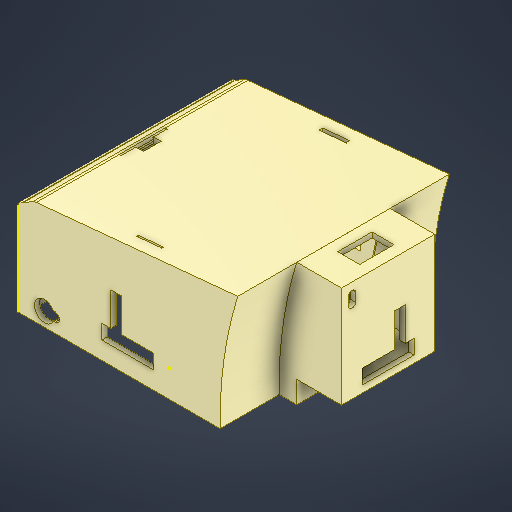
# Autodesk Inventor part: Tapa V.2
Saved by Autodesk Inventor 2026.2 (Build 302298010, 298A)
## iProperties
Created: 2026-05-06
Part Number: Tapa V.2
Material: Genérico
Document SubType Name: Modeling
Designer: migue
Density: 1 g/cm^3
Appearance: Nilón 6
Author: migue
Autodesk Inventor part; units mm, degrees
ref_plane "YZ Plane" through (0, 0, 0) normal (1, 0, 0) x (0, 1, 0)
ref_plane "XZ Plane" through (0, 0, 0) normal (0, 1, 0) x (-1, 0, 0)
sketch "Boceto1" plane through (0, 0, 0) normal (0, 1, 0) x (-1, 0, 0)
  line L0 (-38.316, 43.1554) -> (-63.666, 43.1554)
  line L1 (-63.666, 43.1554) -> (-63.666, -9.8446)
  line L2 (-63.666, -9.8446) -> (-38.316, -9.8446)
  line L3 (-72.7588, 16.6554) -> (45.2156, 16.6554) construction
  line L4 (-38.316, 76.6554) -> (86.334, 76.6554)
  line L5 (86.334, 76.6554) -> (86.334, -43.3446)
  line L6 (86.334, -43.3446) -> (-38.316, -43.3446)
  line L7 (-38.316, -43.3446) -> (-38.316, -9.8446)
  line L8 (-38.316, 43.1554) -> (-38.316, 76.6554)
  circle A0 centre (-42.216, 33.1554) radius 1.65
  circle A1 centre (-42.216, 0.1554) radius 1.65
  line L9 (83.334, 73.6554) -> (-35.316, 73.6554)
  line L10 (-35.316, -40.3446) -> (83.334, -40.3446)
  line L11 (83.334, -40.3446) -> (83.334, 73.6554)
  line L12 (-35.316, 73.6554) -> (-35.316, -40.3446)
  point P0 (-63.666, 16.6554)
  point P1 (-63.666, 16.6554)
  dimension "d5" = 53
  dimension "d6" = 120
  dimension "d7" = 124.65
  dimension "d8" = 25.35
  dimension "d9" = 33.5
  dimension "d10" = 3.3
  dimension "d11" = 16.5
  dimension "d12" = 3.9
  dimension "d13" = 3
  constraints: 26 end point, 6 parallel, 3 horizontal, 3 perpendicular, 2 centre point, 1 coincident, 1 midpoint, 1 symmetric about line, 1 vertical, 2 other
  measures "d5" distance of L2.start L0.end
  measures "d6" distance of L5.start L6.start
  measures "d7" distance of L6.start L7.start
  measures "d8" distance of L2.start L7.end
  measures "d9" distance between parallel lines of L0 L4
  measures "d10" diameter of A0
  measures "d11" distance from line of L3 A0.centre
  measures "d12" distance from line of A0.centre L8
  measures "d13" distance between parallel lines of L4 L9
extrude "Extrusión9" add sketch "Boceto1" against normal blind 3
sketch "Boceto4" plane through (0, 0, 0) normal (0, 1, 0) x (1, 0, 0)
  line L0 (-86.334, 43.3446) -> (38.316, 43.3446) projected
  line L1 (38.316, 43.3446) -> (-86.334, 43.3446)
  line L2 (-86.334, 43.3446) -> (-86.334, -76.6554)
  line L3 (-86.334, -76.6554) -> (38.316, -76.6554)
  line L4 (63.666, 9.8446) -> (63.666, -43.1554) projected
  line L5 (63.666, 9.8446) -> (38.316, 9.8446)
  line L6 (38.316, -43.1554) -> (63.666, -43.1554)
  line L7 (63.666, -43.1554) -> (63.666, 9.8446)
  line L8 (38.316, -76.6554) -> (38.316, -43.1554)
  line L9 (38.316, 9.8446) -> (38.316, 43.3446)
  line L10 (35.316, 6.8446) -> (60.666, 6.8446)
  line L11 (60.666, 6.8446) -> (60.666, -40.1554)
  line L12 (60.666, -40.1554) -> (35.316, -40.1554)
  line L13 (35.316, -40.1554) -> (35.316, -73.6554)
  line L14 (35.316, -73.6554) -> (-83.334, -73.6554)
  line L15 (-83.334, -73.6554) -> (-83.334, 40.3446)
  line L16 (-83.334, 40.3446) -> (35.316, 40.3446)
  line L17 (35.316, 40.3446) -> (35.316, 6.8446)
  point P0 (0, 0)
  dimension "d35" = 3
  constraints: 32 end point, 8 parallel, 2 horizontal, 2 perpendicular, 7 other
  measures "d35" distance between parallel lines of L5 L10
extrude "Extrusión10" add sketch "Boceto4" along normal blind 51.5
sketch "Boceto5" plane through (0, -3, 0) normal (0, -1, 0) x (1, 0, 0)
  line L0 (-86.334, 76.6554) -> (-86.334, -43.3446) projected
  line L1 (38.316, 43.1554) -> (38.316, 76.6554) projected
  line L2 (-86.334, -43.3446) -> (38.316, -43.3446)
  line L3 (38.316, -43.3446) -> (38.316, 76.6554)
  line L4 (38.316, 76.6554) -> (-86.334, 76.6554)
  line L5 (-86.334, 76.6554) -> (-86.334, -43.3446)
  line L6 (35.316, -40.3446) -> (-83.334, -40.3446)
  line L7 (-83.334, -40.3446) -> (-83.334, 73.6554)
  line L8 (-83.334, 73.6554) -> (35.316, 73.6554)
  line L9 (35.316, 73.6554) -> (35.316, -40.3446)
  point P0 (0, 0)
  dimension "d38" = 3
  constraints: 16 end point, 4 parallel, 2 perpendicular, 1 horizontal, 3 other
  measures "d38" distance between parallel lines of L2 L6
extrude "Extrusión11" add sketch "Boceto5" along normal blind 12.5
sketch "Boceto6" plane through (-86.334, 51.5, 76.6554) normal (0, 0, 1) x (1, 0, 0)
  line L0 (0, -67) -> (0, 0) projected
  line L1 (124.65, -67) -> (0, -67) projected
  line L2 (0, 0) -> (124.65, 0)
  line L3 (124.65, 0) -> (124.65, -67)
  line L4 (124.65, -67) -> (0, -67)
  line L5 (0, -67) -> (0, -14.7251)
  line L6 (124.65, 0) -> (2.7125, -11.7389)
  arc A0 (2.7125, -11.7389) -> (0, -14.7251) centre (3, -14.7251) ccw
  line L7 (0, -14.7251) -> (0, 0)
  point P0 (86.334, -51.5)
  point P1 (0, -12)
  dimension "d41" = 55
  dimension "d42" = 3
  constraints: 12 end point, 3 point on line, 3 tangent, 2 parallel, 2 point on circle, 1 centre point, 1 collinear, 1 horizontal, 1 perpendicular
  measures "d41" distance of L0.start point (0, -12)
  measures "d42" radius of A0
extrude "Extrusión12" cut sketch "Boceto6" against normal through all contours L0 L2 L6 A0
sketch "Boceto7" plane through (-86.334, -15.5, 76.6554) normal (0, 0, 1) x (1, 0, 0)
  line L0 (0, 0) -> (0, 52.2749) projected
  point P0 (86.334, 15.5)
sketch "Boceto8" plane through (-86.334, -15.5, 76.6554) normal (0, 0, 1) x (1, 0, 0)
  line L0 (3, 55.2888) -> (124.65, 67)
  line L1 (9.2648, 58.9058) -> (124.65, 70.0139)
  line L2 (3, 55.2888) -> (9.2648, 58.9058)
  line L3 (3, 55.2888) -> (10.234, 55.2888) construction
  line L4 (124.65, 67) -> (124.65, 70.0139)
  point P0 (86.334, 15.5)
  dimension "d46" = 3
  dimension "d47" = 30
  constraints: 10 end point, 1 equal length, 1 horizontal, 1 parallel, 1 vertical
  measures "d46" distance between parallel lines of L0 L1
  measures "d47" angle of L3 L2
extrude "Extrusión13" add sketch "Boceto8" against normal up to surface (120 mm away)
fillet "Empalme1" radius 5 1 edges at (-77.0692, 43.4058, 16.6554)
sketch "Boceto9" plane through (0, 51.5, 0) normal (0, 1, 0) x (1, 0, 0)
  line L0 (63.666, -43.1554) -> (38.316, -43.1554) projected
  line L1 (38.316, 43.3446) -> (38.316, -76.6554) projected
  line L2 (63.666, -43.1554) -> (38.316, -43.1554)
  line L3 (38.316, -43.1554) -> (38.316, 9.7349)
  line L4 (38.316, 9.7349) -> (63.666, 9.7349)
  line L5 (63.666, 9.7349) -> (63.666, -43.1554)
  point P0 (0, 0)
  constraints: 8 end point, 2 parallel, 1 horizontal, 1 perpendicular, 1 point on line
extrude "Extrusión14" add sketch "Boceto9" along normal blind 3
sketch "Boceto10" plane through (38.316, -15.5, -43.3446) normal (0, 0, -1) x (-1, 0, 0)
  line L0 (77.075, 18.25) -> (47.575, 18.25)
  line L1 (47.575, 18.25) -> (47.575, 10)
  line L2 (47.575, 10) -> (77.075, 10)
  line L3 (77.075, 10) -> (77.075, 18.25)
  line L4 (124.65, 0) -> (0, 0) projected
  line L5 (0, 0) -> (124.65, 0) construction
  point P0 (38.316, 15.5)
  point P1 (62.325, 0)
  point P2 (62.325, 10)
  dimension "d53" = 29.5
  dimension "d54" = 8.25
  dimension "d55" = 10
  constraints: 10 end point, 2 horizontal, 2 midpoint, 2 parallel, 1 perpendicular, 1 vertical alignment
  measures "d53" distance of L2.end L1.end
  measures "d54" distance of L1.end L0.end
  measures "d55" distance between parallel lines of L2 L4
extrude "Extrusión15" cut sketch "Boceto10" against normal through all
sketch "Boceto15" plane through (38.316, -15.5, 76.6554) normal (1, 0, 0) x (0, 0, -1)
  line L0 (0, 0) -> (0, 52.2749) construction
  line L1 (120, 0) -> (120, 70.0139) construction
  line L2 (0, 0) -> (120, 0) construction
  line L3 (117, 0) -> (3, 0) construction
  line L4 (57.5, 0) -> (62.5, 0)
  line L5 (62.5, 0) -> (62.5, 5)
  line L6 (62.5, 5) -> (57.5, 5)
  line L7 (57.5, 5) -> (57.5, 0)
  point P0 (76.6554, 15.5)
  point P1 (60, 0)
  dimension "d67" = 5
  dimension "d68" = 5
  constraints: 10 end point, 2 horizontal, 2 midpoint, 2 parallel, 1 perpendicular, 1 point on line
  measures "d67" distance of L6.end L5.end
  measures "d68" distance of L5.end L4.end
extrude "Extrusión17" cut sketch "Boceto15" against normal blind 6
sketch "Boceto16" plane through (38.316, 54.5139, 76.6554) normal (-0.0958265, 0.995398, 0) x (0.995398, 0.0958265, 0)
  line L0 (-6.7092, 120) -> (0, 120) construction
  line L1 (-114.833, 0) -> (-114.833, 120) construction
  line L2 (0, 120) -> (-114.833, 120) construction
  line L3 (-114.833, 120) -> (-114.833, 0) construction
  line L4 (-114.833, 0) -> (0, 0) construction
  line L5 (0, 0) -> (0, 120) construction
  line L6 (-113.633, 73) -> (-114.833, 73)
  line L7 (-114.833, 73) -> (-114.833, 47)
  line L8 (-114.833, 47) -> (-113.633, 47)
  line L9 (-108.833, 65) -> (-113.633, 65)
  line L10 (-113.633, 55) -> (-108.833, 55)
  line L11 (-108.833, 55) -> (-108.833, 65)
  line L12 (-113.633, 47) -> (-113.633, 55)
  line L13 (-113.633, 65) -> (-113.633, 73)
  line L14 (-113.633, 65) -> (-113.633, 55)
  point P0 (-43.3635, 76.6554)
  point P1 (-113.833, 60)
  point P2 (-114.833, 60)
  dimension "d71" = 1.2
  dimension "d72" = 26
  dimension "d75" = 6
  dimension "d76" = 10
  constraints: 26 end point, 7 parallel, 3 horizontal, 2 equal length, 2 midpoint, 2 perpendicular, 1 vertical
  measures "d71" distance of L8.end L7.end
  measures "d72" distance of L7.end L6.end
  measures "d75" distance between parallel lines of L7 L11
  measures "d76" distance between parallel lines of L10 L9
extrude "Extrusión18" cut sketch "Boceto16" against normal blind 2 contours L13 L14 L12 L8 L7 L6
extrude "Extrusión19" cut sketch "Boceto16" against normal blind 4 contours L9 L11 L10 L14
sketch "Boceto17" plane through (0, 54.5, 0) normal (0, 1, 0) x (1, 0, 0)
  line L0 (44.741, -26.4054) -> (57.241, -26.4054)
  line L1 (57.241, -26.4054) -> (57.241, -6.9054)
  line L2 (57.241, -6.9054) -> (44.741, -6.9054)
  line L3 (44.741, -6.9054) -> (44.741, -26.4054)
  line L4 (63.666, 9.8446) -> (63.666, -43.1554) projected
  line L5 (63.666, -43.1554) -> (63.666, 9.8446)
  line L6 (63.666, 9.7349) -> (38.316, 9.7349) projected
  point P0 (0, 0)
  point P1 (50.991, -6.9054)
  point P2 (50.991, 9.7349)
  point P3 (63.666, -16.6554)
  point P4 (57.241, -16.6554)
  dimension "d81" = 12.5
  dimension "d82" = 19.5
  constraints: 10 end point, 4 midpoint, 3 equal length, 1 horizontal, 1 horizontal alignment, 1 perpendicular, 1 vertical alignment
  measures "d81" distance of L2.end L1.end
  measures "d82" distance of L0.end L1.end
extrude "Extrusión20" cut sketch "Boceto17" against normal blind 4
sketch "Boceto18" plane through (63.666, -3, 43.1554) normal (1, 0, 0) x (0, 0, -1)
  line L0 (41.25, 12.25) -> (11.75, 12.25)
  line L1 (11.75, 12.25) -> (11.75, 4)
  line L2 (11.75, 4) -> (41.25, 4)
  line L3 (41.25, 4) -> (41.25, 12.25)
  line L4 (53, 0) -> (0, 0) projected
  point P0 (43.1554, 3)
  point P1 (-15.1668, 30.7927)
  point P2 (71.1672, 15.2927)
  point P3 (26.5, 15.2927)
  point P4 (26.5, 4)
  point P5 (26.5, 0)
  dimension "d85" = 29.5
  dimension "d86" = 8.25
  dimension "d87" = 4
  constraints: 8 end point, 2 midpoint, 2 parallel, 2 vertical alignment, 1 horizontal, 1 perpendicular
  measures "d85" distance of L2.end L1.end
  measures "d86" distance of L1.end L0.end
  measures "d87" distance between parallel lines of L4 L2
extrude "Extrusión21" cut sketch "Boceto18" against normal blind 4
sketch "Boceto19" plane through (38.316, -15.5, -43.3446) normal (0, 0, -1) x (-1, 0, 0)
  line L0 (77.075, 18.25) -> (47.575, 18.25) construction
  line L1 (58.475, 30.446) -> (66.175, 30.446) construction
  line L2 (66.175, 30.446) -> (66.175, 18.25) construction
  line L3 (66.175, 18.25) -> (58.475, 18.25) construction
  line L4 (58.475, 18.25) -> (58.475, 30.446) construction
  line L5 (66.175, 18.25) -> (71.975, 18.25)
  line L6 (71.975, 18.25) -> (71.975, 37.25)
  line L7 (71.975, 37.25) -> (66.175, 37.25)
  line L8 (66.175, 37.25) -> (66.175, 18.25)
  point P0 (38.316, 15.5)
  point P1 (62.325, 18.25)
  point P2 (62.325, 18.25)
  dimension "d90" = 7.7
  dimension "d91" = 5.8
  dimension "d92" = 19
  constraints: 16 end point, 4 parallel, 2 horizontal, 2 midpoint, 2 perpendicular, 1 coincident, 1 point on line
  measures "d90" distance of L2.end L3.end
  measures "d91" distance of L7.end L6.end
  measures "d92" distance of L6.end L5.end
extrude "Extrusión22" cut sketch "Boceto19" against normal through all
sketch "Boceto20" plane through (63.666, -3, 43.1554) normal (1, 0, 0) x (0, 0, -1)
  line L0 (22.65, 17.9725) -> (30.35, 17.9725) construction
  line L1 (30.35, 17.9725) -> (30.35, 12.25) construction
  line L2 (30.35, 12.25) -> (22.65, 12.25) construction
  line L3 (22.65, 12.25) -> (22.65, 17.9725) construction
  line L4 (11.75, 12.25) -> (41.25, 12.25) construction
  line L5 (30.35, 23.0216) -> (30.35, 12.25) construction
  line L6 (30.35, 12.25) -> (36.15, 12.25)
  line L7 (36.15, 12.25) -> (36.15, 31.25)
  line L8 (36.15, 31.25) -> (30.35, 31.25)
  line L9 (30.35, 31.25) -> (30.35, 12.25)
  point P0 (43.1554, 3)
  point P1 (26.5, 12.25)
  point P2 (41.6757, 10.8256)
  point P3 (26.9257, 10.8256)
  point P4 (26.9257, 10.8256)
  dimension "d95" = 7.7
  dimension "d96" = 5.8
  dimension "d97" = 19
  constraints: 18 end point, 4 parallel, 2 horizontal, 2 midpoint, 2 perpendicular, 1 coincident
  measures "d95" distance of L1.end L2.end
  measures "d96" distance of L8.end L7.end
  measures "d97" distance of L7.end L6.end
extrude "Extrusión23" cut sketch "Boceto20" against normal blind 5
sketch "Boceto21" plane through (38.316, 54.5139, 76.6554) normal (-0.0958265, 0.995398, 0) x (0.995398, 0.0958265, 0)
  line L0 (0, 0) -> (0, 120) construction
  line L1 (0, 0) -> (-114.833, 0) construction
  line L2 (0, 120) -> (-114.833, 120) construction
  line L3 (-114.833, 120) -> (-114.833, 0) construction
  line L4 (-114.833, 0) -> (0, 0) construction
  line L5 (0, 0) -> (0, 120) construction
  line L6 (-111.833, 117) -> (-3, 117) construction
  line L7 (-3, 117) -> (-3, 3) construction
  line L8 (-3, 3) -> (-111.833, 3) construction
  line L9 (-111.833, 3) -> (-111.833, 117) construction
  line L10 (-49.7165, 113) -> (-65.1165, 113)
  line L11 (-65.1165, 113) -> (-65.1165, 110.9)
  line L12 (-65.1165, 110.9) -> (-49.7165, 110.9)
  line L13 (-49.7165, 110.9) -> (-49.7165, 113)
  line L14 (-50.2415, 8) -> (-64.5915, 8)
  line L15 (-64.5915, 8) -> (-64.5915, 7)
  line L16 (-64.5915, 7) -> (-50.2415, 7)
  line L17 (-50.2415, 7) -> (-50.2415, 8)
  point P0 (-43.3635, 76.6554)
  point P1 (-57.4165, 117)
  point P2 (-57.4165, 113)
  point P3 (-57.4165, 3)
  point P4 (-57.4165, 7)
  dimension "d100" = 3
  dimension "d101" = 15.4
  dimension "d102" = 2.1
  dimension "d103" = 4
  dimension "d104" = 14.35
  dimension "d105" = 1
  dimension "d106" = 4
  constraints: 32 end point, 8 parallel, 4 midpoint, 4 perpendicular, 3 horizontal, 2 vertical alignment, 3 other
  measures "d100" distance between parallel lines of L2 L6
  measures "d101" distance of L12.end L11.end
  measures "d102" distance of L11.end L10.end
  measures "d103" distance between parallel lines of L6 L10
  measures "d104" distance of L16.end L15.end
  measures "d105" distance of L15.end L14.end
  measures "d106" distance between parallel lines of L8 L16
extrude "Extrusión24" cut sketch "Boceto21" against normal blind 5
sketch "Boceto22" plane through (-86.334, -15.5, -43.3446) normal (-1, 0, 0) x (0, 0, 1)
  circle A0 centre (47.2, 26.1375) radius 8
  circle A1 centre (72.8, 26.1375) radius 8
  line L0 (120, 0) -> (120, 52.2749) projected
  line L1 (47.2, 26.1375) -> (72.8, 26.1375) construction
  line L2 (120, 0) -> (0, 0) construction
  point P0 (43.3446, 15.5)
  point P1 (75.1, 26.1375)
  point P2 (33.5, 26.1375)
  point P3 (120, 26.1375)
  point P4 (60, 26.1375)
  point P5 (60, 0)
  dimension "d109" = 16
  dimension "d110" = 16
  dimension "d112" = 25.6
  constraints: 3 horizontal alignment, 3 midpoint, 2 centre point, 2 end point, 1 horizontal, 1 vertical alignment
  measures "d109" diameter of A0
  measures "d110" diameter of A1
  measures "d112" distance of L1.start L1.end
extrude "Extrusión25" cut sketch "Boceto22" against normal blind 5
sketch "Boceto23" plane through (63.666, -3, 43.1554) normal (1, 0, 0) x (0, 0, -1)
  line L0 (8, 51.4949) -> (7.9873, 46.4949)
  line L1 (3.9873, 46.5051) -> (4, 51.5051)
  arc A0 (8, 51.4949) -> (4, 51.5051) centre (6, 51.5) ccw
  arc A1 (3.9873, 46.5051) -> (7.9873, 46.4949) centre (5.9873, 46.5) ccw
  line L2 (0, 57.5) -> (0, 0) projected
  line L3 (0, 57.5) -> (52.8904, 57.5) projected
  point P0 (43.1554, 3)
  point P1 (3.9937, 49.0051)
  point P2 (7.9937, 48.9949)
  point P3 (12.7392, 43.2596)
  point P4 (12.7392, 43.2596)
  point P5 (13.1216, 48.9949)
  dimension "d115" = 5
  dimension "d116" = 4
  dimension "d117" = 4
  dimension "d118" = 2
  dimension "d119" = 6
  dimension "d120" = 6
  constraints: 4 end point, 4 point on circle, 2 centre point, 2 midpoint, 2 tangent, 1 coincident, 1 horizontal alignment, 1 parallel
  measures "d115" distance of A1.centre A0.centre
  measures "d116" distance of point (3.994, 49.005) point (7.994, 48.995)
  measures "d117" distance between parallel lines of L0 L1
  measures "d118" radius of A0
  measures "d119" distance from line of L2 A0.centre
  measures "d120" distance from line of L3 A0.centre
extrude "Extrusión26" cut sketch "Boceto23" against normal blind 5
sketch "Boceto24" plane through (38.316, -15.5, -43.3446) normal (0, 0, -1) x (-1, 0, 0)
  arc A0 (10, 0) -> (0, 70.0139) centre (-211.5383, 4.079) ccw
  arc A1 (13.0005, 0) -> (3.2357, 69.7024) centre (-211.5383, 4.079) ccw
  line L0 (0, 70.0139) -> (114.3045, 59.0098) projected
  line L1 (124.65, 0) -> (0, 0) projected
  line L2 (0, 0) -> (13.0005, 0)
  line L3 (0, 70.0139) -> (3.2357, 69.7024)
  line L4 (0, 0) -> (0, 70.0139)
  point P0 (-182.8937, 8.158)
  dimension "d126" = 10
  dimension "d127" = 3
  constraints: 6 end point, 4 point on circle, 2 centre point, 2 collinear, 2 point on line, 1 perpendicular
  measures "d126" distance of L1.end A0.start
  measures "d127" radial gap between concentric circles of A0 A1
extrude "Extrusión27" cut sketch "Boceto24" against normal blind 33.5 contours L1 L4 A0
extrude "Extrusión28" add sketch "Boceto24" against normal blind 33.5 contours A0 L0 A1 L1
ref_plane "Plano de trabajo1" through (-86.334, -15.5, 16.6554) normal (0, 0, -1) x (-1, 0, 0)
mirror "Simetría1" about plane through (-86.334, -15.5, 16.6554) normal (0, 0, -1) of "Extrusión27", "Extrusión28"
sketch "Boceto25" plane through (38.316, -3, 43.1554) normal (0, 0, 1) x (1, 0, 0)
  point P0 (-38.316, 3)
sketch "Boceto26" plane through (38.316, -3, 43.1554) normal (0, 0, 1) x (1, 0, 0)
  line L0 (25.35, 57.5) -> (0, 57.5) projected
  line L1 (-10, -12.5) -> (-124.65, -12.5) projected
  arc A0 (0, 57.5) -> (-10, -12.5) centre (211.4033, -8.4148) ccw
  line L2 (-3, -12.5) -> (0, -12.5) projected
  line L3 (-10, -12.5) -> (0, -12.5)
  line L4 (0, -12.5) -> (0, 57.5)
  point P0 (-38.316, 3)
  constraints: 4 end point, 2 point on circle, 1 centre point, 1 horizontal, 1 perpendicular
extrude "Extrusión29" add sketch "Boceto26" against normal blind 3
mirror "Simetría2" about plane through (-86.334, -15.5, 16.6554) normal (0, 0, -1) of "Extrusión29"
sketch "Boceto27" plane through (-86.334, -15.5, 76.6554) normal (0, 0, 1) x (1, 0, 0)
  line L0 (0, 0) -> (0, 52.2749) construction
  line L1 (0, 0) -> (110.5422, 0) construction
  line L2 (110.5422, 0) -> (110.5422, 52.2749) construction
  line L3 (110.5422, 52.2749) -> (0, 52.2749) construction
  line L4 (0, 52.2749) -> (0, 0) construction
  arc A0 (20.1536, 10.55) -> (20.1536, 5.45) centre (15, 8) ccw
  line L5 (9, 14) -> (23.6, 14) construction
  line L6 (23.6, 14) -> (23.6, 2) construction
  line L7 (23.6, 2) -> (9, 2) construction
  line L8 (9, 2) -> (9, 14) construction
  arc A1 (23.6, 8) -> (21.05, 10.55) centre (21.05, 8) ccw construction
  arc A2 (21.05, 5.45) -> (23.6, 8) centre (21.05, 8) ccw construction
  line L9 (21.05, 10.55) -> (20.1536, 10.55)
  line L10 (21.05, 5.45) -> (20.1536, 5.45)
  arc A3 (21.05, 5.45) -> (21.05, 10.55) centre (21.05, 8) ccw
  point P0 (86.334, 15.5)
  point P1 (21.05, 10.55)
  dimension "d134" = 11.5
  dimension "d135" = 15
  dimension "d136" = 8
  dimension "d137" = 14.6
  dimension "d138" = 2.55
  constraints: 20 end point, 9 point on circle, 5 parallel, 4 centre point, 3 coincident, 3 horizontal, 2 perpendicular, 1 concentric, 1 midpoint
  measures "d134" diameter of A0
  measures "d135" distance from line of L0 A0.centre
  measures "d136" distance from line of L1 A0.centre
  measures "d137" distance of L6.end L7.end
  measures "d138" distance of A1.start point (21.05, 8)
extrude "Extrusión30" cut sketch "Boceto27" against normal through all
